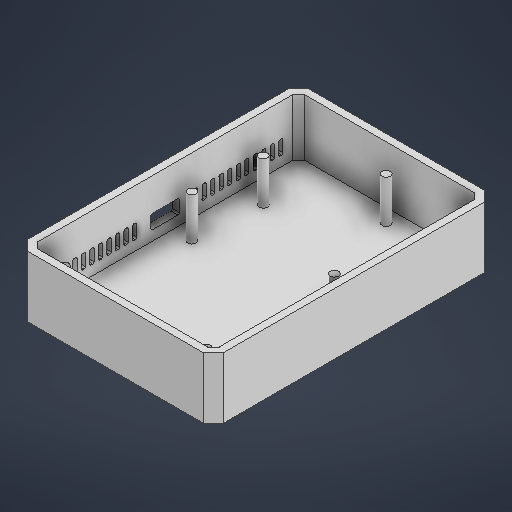
# Autodesk Inventor part: test1
Saved by Autodesk Inventor 2025.1 (Build 291241000, 241)
## iProperties
Created: 2025-05-05
Part Number: test1
Material: Типовые
Document SubType Name: Modeling
Designer: bogda
Density: 1 g/cm^3
Appearance: По умолчанию
Author: bogda
Autodesk Inventor part; units mm, degrees
ref_plane "YZ Plane" through (0, 0, 0) normal (1, 0, 0) x (0, 1, 0)
ref_plane "XZ Plane" through (0, 0, 0) normal (0, 1, 0) x (-1, 0, 0)
ref_plane "XY Plane" through (0, 0, 0) normal (0, 0, 1) x (1, 0, 0)
sketch "Эскиз1" plane through (0, 0, 0) normal (0, 1, 0) x (-1, 0, 0)
  line L0 (30, 45) -> (-30, 45)
  line L1 (-30, 45) -> (-30, -45)
  line L2 (-30, -45) -> (30, -45)
  line L3 (30, -45) -> (30, 45)
  line L4 (30, 45) -> (-30, -45) construction
  line L5 (-30, 45) -> (30, -45) construction
  line L6 (30, 45) -> (24.95, 45)
  circle A0 centre (24.95, 42.45) radius 1.5
  line L7 (-30, 45) -> (-24.95, 45)
  circle A1 centre (-24.95, 42.45) radius 1.5
  circle A2 centre (25.2371, -2.6491) radius 1.5
  circle A3 centre (-24.95, -2.65) radius 1.5
  circle A4 centre (23.5871, -26.1691) radius 1.5
  circle A5 centre (-3.6129, -42.2191) radius 1.5
  line L8 (30, 47) -> (32, 45)
  line L9 (-32, -45) -> (-30, -47)
  line L10 (32, -45) -> (30, -47)
  line L11 (-32, 45) -> (-30, 47)
  line L12 (32, 45) -> (32, -45)
  line L13 (30, -47) -> (-30, -47)
  line L14 (-32, 45) -> (-32, -45)
  line L15 (30, 47) -> (-30, 47)
  line L16 (-31.0355, 49.5) -> (-34.5, 46.0355)
  line L17 (-34.5, 46.0355) -> (-34.5, -46.0355)
  line L18 (-34.5, -46.0355) -> (-31.0355, -49.5)
  line L19 (-31.0355, -49.5) -> (31.0355, -49.5)
  line L20 (31.0355, -49.5) -> (34.5, -46.0355)
  line L21 (34.5, -46.0355) -> (34.5, 46.0355)
  line L22 (34.5, 46.0355) -> (31.0355, 49.5)
  line L23 (31.0355, 49.5) -> (-31.0355, 49.5)
  point P0 (0, 0)
  dimension "d4" = 3
  dimension "d7" = 3
  dimension "d9" = 3
  dimension "d11" = 3
  dimension "d14" = 3
  dimension "d17" = 3
  dimension "d22" = 2
  dimension "d26" = 2
  dimension "d27" = 2.5
  constraints: 48 end point, 6 centre point, 2 horizontal, 2 midpoint, 2 parallel, 2 point on line, 1 perpendicular, 7 other
  measures "d4" diameter of A0
  measures "d7" diameter of A1
  measures "d9" diameter of A2
  measures "d11" diameter of A3
  measures "d14" diameter of A4
  measures "d17" diameter of A5
  measures "d22" distance of L2.end L10.end
  measures "d26" distance of L0.end L11.start
  measures "d27" distance between parallel lines of L15 L23
extrude "Выдавливание1" add sketch "Эскиз1" against normal blind 1.5 contours L3 L2 L1 L0 | A0 | A1 | A2 | A3 | A4 | A5 | L8 L12 L10 L13 L9 L14 L11 L15 | L23 L22 L21 L20 L19 L18 L17 L16
extrude "Выдавливание2" add sketch "Эскиз1" along normal blind 20 contours L23 L22 L21 L20 L19 L18 L17 L16
extrude "Выдавливание3" add sketch "Эскиз1" along normal blind 15 contours A0 | A1 | A2 | A3 | A4 | A5
sketch "Эскиз2" plane through (-34.5, -1.5, -46.0355) normal (-1, 0, 0) x (0, 0, 1)
  line L0 (-3.4645, 0) -> (-3.4645, 21.5) projected
  line L1 (0, 0) -> (92.0711, 0) projected
  line L2 (46.0355, 5) -> (50.5355, 5)
  line L3 (51.0355, 5.5) -> (51.0355, 9.5)
  line L4 (50.5355, 10) -> (41.5355, 10)
  line L5 (41.0355, 9.5) -> (41.0355, 5.5)
  line L6 (41.5355, 5) -> (46.0355, 5)
  arc A0 (41.5355, 10) -> (41.0355, 9.5) centre (41.5355, 9.5) ccw
  arc A1 (41.0355, 5.5) -> (41.5355, 5) centre (41.5355, 5.5) ccw
  arc A2 (50.5355, 5) -> (51.0355, 5.5) centre (50.5355, 5.5) ccw
  arc A3 (51.0355, 9.5) -> (50.5355, 10) centre (50.5355, 9.5) ccw
  line L7 (56.0355, 5.5) -> (56.0355, 5.5)
  line L8 (56.5355, 5) -> (57.0355, 5)
  line L9 (57.5355, 5.5) -> (57.5355, 9.5)
  line L10 (57.0355, 10) -> (56.5355, 10)
  line L11 (56.0355, 9.5) -> (56.0355, 5.5)
  arc A4 (56.5355, 10) -> (56.0355, 9.5) centre (56.5355, 9.5) ccw
  arc A5 (57.5355, 9.5) -> (57.0355, 10) centre (57.0355, 9.5) ccw
  arc A6 (56.0355, 5.5) -> (56.5355, 5) centre (56.5355, 5.5) ccw
  arc A7 (57.0355, 5) -> (57.5355, 5.5) centre (57.0355, 5.5) ccw
  line L12 (59.0355, 5.9277) -> (59.0355, 9.5)
  line L13 (59.5355, 10) -> (60.0355, 10)
  line L14 (62.0355, 5.9277) -> (62.0355, 9.5)
  line L15 (62.5355, 10) -> (63.0355, 10)
  line L16 (63.5355, 9.5) -> (63.5355, 5.5)
  line L17 (63.0355, 5) -> (62.5355, 5)
  line L18 (62.0355, 5.5) -> (62.0355, 5.9277)
  line L19 (59.0355, 10) -> (59.0355, 5.5)
  line L20 (59.5355, 5) -> (60.0355, 5)
  line L21 (60.5355, 5.5) -> (60.5355, 9.5)
  line L22 (65.0355, 5.9277) -> (65.0355, 5.5)
  line L23 (65.5355, 5) -> (66.0355, 5)
  line L24 (66.5355, 5.5) -> (66.5355, 9.5)
  line L25 (66.0355, 10) -> (65.5355, 10)
  line L26 (65.0355, 9.5) -> (65.0355, 5.9277)
  line L27 (68.0355, 5.9277) -> (68.0355, 5.5)
  line L28 (68.5355, 5) -> (69.0411, 5)
  line L29 (69.5411, 5.4944) -> (69.5858, 9.4944)
  line L30 (69.0858, 10) -> (68.5355, 10)
  line L31 (68.0355, 5.9277) -> (68.0355, 9.5)
  arc A8 (59.5355, 10) -> (59.0355, 9.5) centre (59.5355, 9.5) ccw
  arc A9 (59.0355, 5.5) -> (59.5355, 5) centre (59.5355, 5.5) ccw
  arc A10 (60.0355, 5) -> (60.5355, 5.5) centre (60.0355, 5.5) ccw
  arc A11 (60.5355, 9.5) -> (60.0355, 10) centre (60.0355, 9.5) ccw
  arc A12 (62.5355, 10) -> (62.0355, 9.5) centre (62.5355, 9.5) ccw
  arc A13 (62.0355, 5.5) -> (62.5355, 5) centre (62.5355, 5.5) ccw
  arc A14 (63.0355, 5) -> (63.5355, 5.5) centre (63.0355, 5.5) ccw
  arc A15 (63.5355, 9.5) -> (63.0355, 10) centre (63.0355, 9.5) ccw
  arc A16 (65.5355, 10) -> (65.0355, 9.5) centre (65.5355, 9.5) ccw
  arc A17 (65.0355, 5.5) -> (65.5355, 5) centre (65.5355, 5.5) ccw
  arc A18 (66.0355, 5) -> (66.5355, 5.5) centre (66.0355, 5.5) ccw
  arc A19 (66.5355, 9.5) -> (66.0355, 10) centre (66.0355, 9.5) ccw
  arc A20 (68.5355, 10) -> (68.0355, 9.5) centre (68.5355, 9.5) ccw
  arc A21 (69.5858, 9.4944) -> (69.0858, 10) centre (69.0858, 9.5) ccw
  arc A22 (69.0411, 5) -> (69.5411, 5.4944) centre (69.0411, 5.5) ccw
  arc A23 (68.0355, 5.5) -> (68.5355, 5) centre (68.5355, 5.5) ccw
  line L32 (71.0355, 5.9277) -> (71.0355, 5.5)
  line L33 (72.5411, 5.4944) -> (72.5858, 9.4944)
  line L34 (72.0858, 10) -> (71.5355, 10)
  line L35 (71.0355, 5.9277) -> (71.0355, 9.5)
  arc A24 (71.5355, 10) -> (71.0355, 9.5) centre (71.5355, 9.5) ccw
  arc A25 (72.5858, 9.4944) -> (72.0858, 10) centre (72.0858, 9.5) ccw
  line L36 (71.5355, 5) -> (72.0411, 5)
  arc A26 (72.0411, 5) -> (72.5411, 5.4944) centre (72.0411, 5.5) ccw
  arc A27 (71.0355, 5.5) -> (71.5355, 5) centre (71.5355, 5.5) ccw
  line L37 (74.0355, 5.9277) -> (74.0355, 5.5)
  line L38 (75.5411, 5.4944) -> (75.5858, 9.4944)
  line L39 (75.0858, 10) -> (74.5355, 10)
  line L40 (74.0355, 5.9277) -> (74.0355, 9.5)
  arc A28 (74.5355, 10) -> (74.0355, 9.5) centre (74.5355, 9.5) ccw
  arc A29 (75.5858, 9.4944) -> (75.0858, 10) centre (75.0858, 9.5) ccw
  line L41 (74.5355, 5) -> (75.0411, 5)
  arc A30 (75.0411, 5) -> (75.5411, 5.4944) centre (75.0411, 5.5) ccw
  arc A31 (74.0355, 5.5) -> (74.5355, 5) centre (74.5355, 5.5) ccw
  line L42 (77.0355, 5.9277) -> (77.0355, 5.5)
  line L43 (78.5411, 5.4944) -> (78.5858, 9.4944)
  line L44 (78.0858, 10) -> (77.5355, 10)
  line L45 (77.0355, 5.9277) -> (77.0355, 9.5)
  arc A32 (77.5355, 10) -> (77.0355, 9.5) centre (77.5355, 9.5) ccw
  arc A33 (78.5858, 9.4944) -> (78.0858, 10) centre (78.0858, 9.5) ccw
  line L46 (77.5355, 5) -> (78.0411, 5)
  arc A34 (78.0411, 5) -> (78.5411, 5.4944) centre (78.0411, 5.5) ccw
  arc A35 (77.0355, 5.5) -> (77.5355, 5) centre (77.5355, 5.5) ccw
  line L47 (80.0355, 5.9277) -> (80.0355, 5.5)
  line L48 (81.5411, 5.4944) -> (81.5858, 9.4944)
  line L49 (81.0858, 10) -> (80.5355, 10)
  line L50 (80.0355, 5.9277) -> (80.0355, 9.5)
  arc A36 (80.5355, 10) -> (80.0355, 9.5) centre (80.5355, 9.5) ccw
  arc A37 (81.5858, 9.4944) -> (81.0858, 10) centre (81.0858, 9.5) ccw
  line L51 (80.5355, 5) -> (81.0411, 5)
  arc A38 (81.0411, 5) -> (81.5411, 5.4944) centre (81.0411, 5.5) ccw
  arc A39 (80.0355, 5.5) -> (80.5355, 5) centre (80.5355, 5.5) ccw
  line L52 (83.0355, 5.9277) -> (83.0355, 5.5)
  line L53 (84.5411, 5.4944) -> (84.5858, 9.4944)
  line L54 (84.0858, 10) -> (83.5355, 10)
  line L55 (83.0355, 5.9277) -> (83.0355, 9.5)
  arc A40 (83.5355, 10) -> (83.0355, 9.5) centre (83.5355, 9.5) ccw
  arc A41 (84.5858, 9.4944) -> (84.0858, 10) centre (84.0858, 9.5) ccw
  line L56 (83.5355, 5) -> (84.0411, 5)
  arc A42 (84.0411, 5) -> (84.5411, 5.4944) centre (84.0411, 5.5) ccw
  arc A43 (83.0355, 5.5) -> (83.5355, 5) centre (83.5355, 5.5) ccw
  line L57 (86.0355, 5.9277) -> (86.0355, 5.5)
  line L58 (87.5411, 5.4944) -> (87.5858, 9.4944)
  line L59 (87.0858, 10) -> (86.5355, 10)
  line L60 (86.0355, 5.9277) -> (86.0355, 9.5)
  arc A44 (86.5355, 10) -> (86.0355, 9.5) centre (86.5355, 9.5) ccw
  arc A45 (87.5858, 9.4944) -> (87.0858, 10) centre (87.0858, 9.5) ccw
  line L61 (86.5355, 5) -> (87.0411, 5)
  arc A46 (87.0411, 5) -> (87.5411, 5.4944) centre (87.0411, 5.5) ccw
  arc A47 (86.0355, 5.5) -> (86.5355, 5) centre (86.5355, 5.5) ccw
  line L62 (36.0355, 6.5654) -> (36.0355, 5.5)
  line L63 (35.5355, 5) -> (35.0355, 5)
  line L64 (34.5355, 5.5) -> (34.5355, 9.5)
  line L65 (35.0355, 10) -> (35.5355, 10)
  line L66 (36.0355, 9.5) -> (36.0355, 6.5654)
  arc A48 (35.0355, 10) -> (34.5355, 9.5) centre (35.0355, 9.5) ccw
  arc A49 (34.5355, 5.5) -> (35.0355, 5) centre (35.0355, 5.5) ccw
  arc A50 (35.5355, 5) -> (36.0355, 5.5) centre (35.5355, 5.5) ccw
  arc A51 (36.0355, 9.5) -> (35.5355, 10) centre (35.5355, 9.5) ccw
  arc A52 (33.0355, 9.5) -> (32.5355, 10) centre (32.5355, 9.5) ccw
  line L67 (33.0355, 9.5) -> (33.0355, 6.5654)
  line L68 (32.0355, 10) -> (32.5355, 10)
  arc A53 (32.0355, 10) -> (31.5355, 9.5) centre (32.0355, 9.5) ccw
  line L69 (33.0355, 6.5654) -> (33.0355, 5.5)
  line L70 (31.5355, 5.5) -> (31.5355, 9.5)
  line L71 (32.5355, 5) -> (32.0355, 5)
  arc A54 (31.5355, 5.5) -> (32.0355, 5) centre (32.0355, 5.5) ccw
  arc A55 (32.5355, 5) -> (33.0355, 5.5) centre (32.5355, 5.5) ccw
  arc A56 (30.0355, 9.5) -> (29.5355, 10) centre (29.5355, 9.5) ccw
  line L72 (30.0355, 9.5) -> (30.0355, 6.5654)
  line L73 (29.0355, 10) -> (29.5355, 10)
  arc A57 (29.0355, 10) -> (28.5355, 9.5) centre (29.0355, 9.5) ccw
  line L74 (30.0355, 6.5654) -> (30.0355, 5.5)
  line L75 (28.5355, 5.5) -> (28.5355, 9.5)
  line L76 (29.5355, 5) -> (29.0355, 5)
  arc A58 (28.5355, 5.5) -> (29.0355, 5) centre (29.0355, 5.5) ccw
  arc A59 (29.5355, 5) -> (30.0355, 5.5) centre (29.5355, 5.5) ccw
  arc A60 (27.0355, 9.5) -> (26.5355, 10) centre (26.5355, 9.5) ccw
  line L77 (27.0355, 9.5) -> (27.0355, 6.5654)
  line L78 (26.0355, 10) -> (26.5355, 10)
  arc A61 (26.0355, 10) -> (25.5355, 9.5) centre (26.0355, 9.5) ccw
  line L79 (27.0355, 6.5654) -> (27.0355, 5.5)
  line L80 (25.5355, 5.5) -> (25.5355, 9.5)
  line L81 (26.5355, 5) -> (26.0355, 5)
  arc A62 (25.5355, 5.5) -> (26.0355, 5) centre (26.0355, 5.5) ccw
  arc A63 (26.5355, 5) -> (27.0355, 5.5) centre (26.5355, 5.5) ccw
  arc A64 (24.0355, 9.5) -> (23.5355, 10) centre (23.5355, 9.5) ccw
  line L82 (24.0355, 9.5) -> (24.0355, 6.5654)
  line L83 (23.0355, 10) -> (23.5355, 10)
  arc A65 (23.0355, 10) -> (22.5355, 9.5) centre (23.0355, 9.5) ccw
  line L84 (24.0355, 6.5654) -> (24.0355, 5.5)
  line L85 (22.5355, 5.5) -> (22.5355, 9.5)
  line L86 (23.5355, 5) -> (23.0355, 5)
  arc A66 (22.5355, 5.5) -> (23.0355, 5) centre (23.0355, 5.5) ccw
  arc A67 (23.5355, 5) -> (24.0355, 5.5) centre (23.5355, 5.5) ccw
  arc A68 (21.0355, 9.5) -> (20.5355, 10) centre (20.5355, 9.5) ccw
  line L87 (21.0355, 9.5) -> (21.0355, 6.5654)
  line L88 (20.0355, 10) -> (20.5355, 10)
  arc A69 (20.0355, 10) -> (19.5355, 9.5) centre (20.0355, 9.5) ccw
  line L89 (21.0355, 6.5654) -> (21.0355, 5.5)
  line L90 (19.5355, 5.5) -> (19.5355, 9.5)
  line L91 (20.5355, 5) -> (20.0355, 5)
  arc A70 (19.5355, 5.5) -> (20.0355, 5) centre (20.0355, 5.5) ccw
  arc A71 (20.5355, 5) -> (21.0355, 5.5) centre (20.5355, 5.5) ccw
  arc A72 (18.0355, 9.5) -> (17.5355, 10) centre (17.5355, 9.5) ccw
  line L92 (18.0355, 9.5) -> (18.0355, 6.5654)
  line L93 (17.0355, 10) -> (17.5355, 10)
  arc A73 (17.0355, 10) -> (16.5355, 9.5) centre (17.0355, 9.5) ccw
  line L94 (18.0355, 6.5654) -> (18.0355, 5.5)
  line L95 (16.5355, 5.5) -> (16.5355, 9.5)
  line L96 (17.5355, 5) -> (17.0355, 5)
  arc A74 (16.5355, 5.5) -> (17.0355, 5) centre (17.0355, 5.5) ccw
  arc A75 (17.5355, 5) -> (18.0355, 5.5) centre (17.5355, 5.5) ccw
  arc A76 (15.0355, 9.5) -> (14.5355, 10) centre (14.5355, 9.5) ccw
  line L97 (15.0355, 9.5) -> (15.0355, 6.5654)
  line L98 (14.0355, 10) -> (14.5355, 10)
  arc A77 (14.0355, 10) -> (13.5355, 9.5) centre (14.0355, 9.5) ccw
  line L99 (15.0355, 6.5654) -> (15.0355, 5.5)
  line L100 (13.5355, 5.5) -> (13.5355, 9.5)
  line L101 (14.5355, 5) -> (14.0355, 5)
  arc A78 (13.5355, 5.5) -> (14.0355, 5) centre (14.0355, 5.5) ccw
  arc A79 (14.5355, 5) -> (15.0355, 5.5) centre (14.5355, 5.5) ccw
  arc A80 (12.0355, 9.5) -> (11.5355, 10) centre (11.5355, 9.5) ccw
  line L102 (12.0355, 9.5) -> (12.0355, 6.5654)
  line L103 (11.0355, 10) -> (11.5355, 10)
  arc A81 (11.0355, 10) -> (10.5355, 9.5) centre (11.0355, 9.5) ccw
  line L104 (12.0355, 6.5654) -> (12.0355, 5.5)
  line L105 (10.5355, 5.5) -> (10.5355, 9.5)
  line L106 (11.5355, 5) -> (11.0355, 5)
  arc A82 (10.5355, 5.5) -> (11.0355, 5) centre (11.0355, 5.5) ccw
  arc A83 (11.5355, 5) -> (12.0355, 5.5) centre (11.5355, 5.5) ccw
  arc A84 (9.0355, 9.5) -> (8.5355, 10) centre (8.5355, 9.5) ccw
  line L107 (9.0355, 9.5) -> (9.0355, 6.5654)
  line L108 (8.0355, 10) -> (8.5355, 10)
  arc A85 (8.0355, 10) -> (7.5355, 9.5) centre (8.0355, 9.5) ccw
  line L109 (9.0355, 6.5654) -> (9.0355, 5.5)
  line L110 (7.5355, 5.5) -> (7.5355, 9.5)
  line L111 (8.5355, 5) -> (8.0355, 5)
  arc A86 (7.5355, 5.5) -> (8.0355, 5) centre (8.0355, 5.5) ccw
  arc A87 (8.5355, 5) -> (9.0355, 5.5) centre (8.5355, 5.5) ccw
  arc A88 (6.0355, 9.5) -> (5.5355, 10) centre (5.5355, 9.5) ccw
  line L112 (6.0355, 9.5) -> (6.0355, 6.5654)
  line L113 (5.0355, 10) -> (5.5355, 10)
  arc A89 (5.0355, 10) -> (4.5355, 9.5) centre (5.0355, 9.5) ccw
  line L114 (6.0355, 6.5654) -> (6.0355, 5.5)
  line L115 (4.5355, 5.5) -> (4.5355, 9.5)
  line L116 (5.5355, 5) -> (5.0355, 5)
  arc A90 (4.5355, 5.5) -> (5.0355, 5) centre (5.0355, 5.5) ccw
  arc A91 (5.5355, 5) -> (6.0355, 5.5) centre (5.5355, 5.5) ccw
  point P0 (46.0355, 1.5)
  point P1 (51.0355, 5)
  point P2 (51.0355, 10)
  point P3 (41.0355, 10)
  point P4 (41.0355, 5)
  point P5 (56.0355, 5)
  point P6 (57.5355, 5)
  point P7 (56.0355, 10)
  point P8 (60.5355, 10)
  point P9 (62.0355, 10)
  point P10 (63.5355, 10)
  point P11 (63.5355, 5)
  point P12 (59.0355, 5)
  point P13 (65.0355, 5)
  point P14 (66.5355, 5)
  point P15 (65.0355, 10)
  point P16 (68.0355, 5)
  point P17 (69.5355, 5)
  point P18 (69.5914, 10)
  point P19 (68.0355, 10)
  point P20 (71.0355, 10)
  point P21 (71.0355, 5)
  point P22 (72.5914, 10)
  point P23 (72.5355, 5)
  point P24 (74.0355, 10)
  point P25 (74.0355, 5)
  point P26 (75.5914, 10)
  point P27 (75.5355, 5)
  point P28 (77.0355, 10)
  point P29 (77.0355, 5)
  point P30 (78.5914, 10)
  point P31 (78.5355, 5)
  point P32 (80.0355, 10)
  point P33 (80.0355, 5)
  point P34 (81.5914, 10)
  point P35 (81.5355, 5)
  point P36 (83.0355, 10)
  point P37 (83.0355, 5)
  point P38 (84.5914, 10)
  point P39 (84.5355, 5)
  point P40 (86.0355, 10)
  point P41 (86.0355, 5)
  point P42 (87.5914, 10)
  point P43 (87.5355, 5)
  point P44 (36.0355, 5)
  point P45 (34.5355, 5)
  point P46 (34.5355, 10)
  point P47 (36.0355, 10)
  point P48 (33.0355, 10)
  point P49 (31.5355, 10)
  point P50 (33.0355, 5)
  point P51 (31.5355, 5)
  point P52 (30.0355, 10)
  point P53 (28.5355, 10)
  point P54 (30.0355, 5)
  point P55 (28.5355, 5)
  point P56 (27.0355, 10)
  point P57 (25.5355, 10)
  point P58 (27.0355, 5)
  point P59 (25.5355, 5)
  point P60 (24.0355, 10)
  point P61 (22.5355, 10)
  point P62 (24.0355, 5)
  point P63 (22.5355, 5)
  point P64 (21.0355, 10)
  point P65 (19.5355, 10)
  point P66 (21.0355, 5)
  point P67 (19.5355, 5)
  point P68 (18.0355, 10)
  point P69 (16.5355, 10)
  point P70 (18.0355, 5)
  point P71 (16.5355, 5)
  point P72 (15.0355, 10)
  point P73 (13.5355, 10)
  point P74 (15.0355, 5)
  point P75 (13.5355, 5)
  point P76 (12.0355, 10)
  point P77 (10.5355, 10)
  point P78 (12.0355, 5)
  point P79 (10.5355, 5)
  point P80 (9.0355, 10)
  point P81 (7.5355, 10)
  point P82 (9.0355, 5)
  point P83 (7.5355, 5)
  point P84 (6.0355, 10)
  point P85 (4.5355, 10)
  point P86 (6.0355, 5)
  point P87 (4.5355, 5)
  point P88 (59.0355, 5.9277)
  point P89 (56.0355, 5.5)
  dimension "d37" = 5
  dimension "d38" = 10
  dimension "d39" = 5
  dimension "d40" = 0.5
  dimension "d41" = 5
  dimension "d42" = 1.5
  dimension "d43" = 0.5
  dimension "d44" = 0.5
  dimension "d50" = 5
  dimension "d52" = 1.5
  dimension "d54" = 1.5
  dimension "d55" = 0.5
  dimension "d58" = 3
  dimension "d64" = 1.5
  dimension "d65" = 5
  dimension "d66" = 0.5
  dimension "d69" = 3
  constraints: 230 end point, 203 point on line, 184 point on circle, 92 centre point, 56 tangent, 23 equal radius, 19 perpendicular, 4 vertical, 2 collinear, 2 horizontal, 415 other
  measures "d37" distance of point (51.036, 5) point (51.036, 10)
  measures "d38" distance of point (51.036, 10) point (41.036, 10)
  measures "d39" distance of point (41.036, 10) point (41.036, 5)
  measures "d40" radius of A0
  measures "d41" distance of L3.start L7.start
  measures "d42" distance of point (56.036, 5) point (57.536, 5)
  measures "d43" radius of A4
  measures "d44" radius of A6
  measures "d50" distance of L19.start point (59.036, 5)
  measures "d52" distance of point (65.036, 5) point (66.536, 5)
  measures "d54" distance of point (68.036, 5) point (69.536, 5)
  measures "d55" radius of A8
  measures "d58" distance of L27.start L32.start
  measures "d64" distance of point (36.036, 5) point (34.536, 5)
  measures "d65" distance of point (34.536, 5) point (34.536, 10)
  measures "d66" radius of A48
  measures "d69" distance of L66.start L67.start
extrude "Выдавливание4" cut sketch "Эскиз2" against normal blind 5
